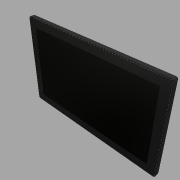
# Autodesk Inventor part: MageDok Screen
Saved by Autodesk Inventor 2019 (Build 230136000, 136)
## iProperties
Created: 2019-02-07
Part Number: MageDok Screen
Material: Generic
Document SubType Name: Modeling
Designer: Ben
Density: 1 g/cm^3
Appearance: Default
Author: Ben
Autodesk Inventor part; units mm, degrees
ref_plane "YZ Plane" through (0, 0, 0) normal (1, 0, 0) x (0, 1, 0)
ref_plane "XZ Plane" through (0, 0, 0) normal (0, 1, 0) x (-1, 0, 0)
sketch "Sketch1" plane through (0, 0, 0) normal (0, 0, 1) x (1, 0, 0)
  line L0 (152.5, -93.75) -> (-152.5, -93.75)
  line L1 (-152.5, -93.75) -> (-152.5, 93.75)
  line L2 (-152.5, 93.75) -> (152.5, 93.75)
  line L3 (152.5, 93.75) -> (152.5, -93.75)
  line L4 (152.5, -93.75) -> (-152.5, 93.75) construction
  line L5 (-152.5, -93.75) -> (152.5, 93.75) construction
  point P0 (0, 0)
  dimension "d0" = 305
  dimension "d1" = 187.5
  constraints: 12 end point, 2 midpoint, 2 parallel, 1 horizontal, 1 perpendicular
  measures "d0" distance of L1.end L2.end
  measures "d1" distance of L0.end L1.end
extrude "Extrusion1" add sketch "Sketch1" along normal blind 10.5
fillet "Fillet1" radius 4 4 edges at (152.5, 93.75, 5.25) (-152.5, 93.75, 5.25) (-152.5, -93.75, 5.25) (152.5, -93.75, 5.25)
chamfer "Chamfer1" distance 0.5 distance2 1 8 edges at (0, 93.75, 10.5) (-151.3284, 92.5784, 10.5) (-152.5, 0, 10.5) (-151.3284, -92.5784, 10.5) (0, -93.75, 10.5) (151.3284, -92.5784, 10.5) (152.5, 0, 10.5) (151.3284, 92.5784, 10.5) measured on face at (49.5, -31.25, 10.5)
chamfer "Chamfer2" distance 0.5 distance2 1.5 8 edges at (0, 93.75, 0) (151.3284, 92.5784, 0) (152.5, 0, 0) (151.3284, -92.5784, 0) (0, -93.75, 0) (-151.3284, -92.5784, 0) (-152.5, 0, 0) (-151.3284, 92.5784, 0) measured on face at (49.5, -31.25, 0)
sketch "Sketch2" plane through (0, 0, 10.5) normal (0, 0, 1) x (1, 0, 0)
  line L0 (-148.5, 93.25) -> (148.5, 93.25) construction
  arc A0 (-148.5, 93.25) -> (-152, 89.75) centre (-148.5, 89.75) ccw construction
  line L1 (-152, -89.75) -> (-152, 89.75) construction
  arc A1 (-152, -89.75) -> (-148.5, -93.25) centre (-148.5, -89.75) ccw construction
  line L2 (148.5, -93.25) -> (-148.5, -93.25) construction
  arc A2 (148.5, -93.25) -> (152, -89.75) centre (148.5, -89.75) ccw construction
  line L3 (152, 89.75) -> (152, -89.75) construction
  arc A3 (152, 89.75) -> (148.5, 93.25) centre (148.5, 89.75) ccw construction
  line L4 (148.5, 92.75) -> (-148.5, 92.75)
  arc A4 (-148.5, 92.75) -> (-151.5, 89.75) centre (-148.5, 89.75) ccw
  line L5 (-151.5, 89.75) -> (-151.5, -89.75)
  arc A5 (-151.5, -89.75) -> (-148.5, -92.75) centre (-148.5, -89.75) ccw
  line L6 (-148.5, -92.75) -> (148.5, -92.75)
  arc A6 (148.5, -92.75) -> (151.5, -89.75) centre (148.5, -89.75) ccw
  line L7 (151.5, -89.75) -> (151.5, 89.75)
  arc A7 (151.5, 89.75) -> (148.5, 92.75) centre (148.5, 89.75) ccw
  point P0 (0, 0)
  dimension "d11" = 0.5
  constraints: 8 end point, 8 point on circle, 4 centre point, 7 other
  measures "d11" distance between parallel lines of L0 L4
extrude "Extrusion2" cut sketch "Sketch2" against normal blind 0.25
fillet "Fillet2" radius 0.25 16 edges at (-150.6213, 91.8713, 10.5) (0, 92.75, 10.5) (150.6213, 91.8713, 10.5) (151.5, 0, 10.5) (150.6213, -91.8713, 10.5) (0, -92.75, 10.5) (-150.6213, -91.8713, 10.5) (-151.5, 0, 10.5) (0, 93.25, 10.5) (-150.9749, 92.2249, 10.5) (-152, 0, 10.5) (-150.9749, -92.2249, 10.5) (0, -93.25, 10.5) (150.9749, -92.2249, 10.5) (152, 0, 10.5) (150.9749, 92.2249, 10.5)
ref_plane "Work Plane1" through (0, 0, 10.5) normal (0, 0, 1) x (1, 0, 0)
sketch "Sketch3" plane through (0, 0, 10.5) normal (0, 0, 1) x (1, 0, 0)
  line L0 (-148.5, 92.75) -> (148.5, 92.75) projected
  arc A0 (-148.5, 92.75) -> (-151.5, 89.75) centre (-148.5, 89.75) ccw projected
  line L1 (-151.5, -89.75) -> (-151.5, 89.75) projected
  arc A1 (-151.5, -89.75) -> (-148.5, -92.75) centre (-148.5, -89.75) ccw projected
  line L2 (148.5, -92.75) -> (-148.5, -92.75) projected
  arc A2 (148.5, -92.75) -> (151.5, -89.75) centre (148.5, -89.75) ccw projected
  line L3 (151.5, 89.75) -> (151.5, -89.75) projected
  arc A3 (151.5, 89.75) -> (148.5, 92.75) centre (148.5, 89.75) ccw projected
  line L4 (-134.5, -75.75) -> (-134.5, 75.75)
  line L5 (-134.5, 75.75) -> (134.5, 75.75)
  line L6 (134.5, 75.75) -> (134.5, -75.75)
  line L7 (134.5, -75.75) -> (-134.5, -75.75)
  point P0 (0, 0)
  dimension "d16" = 17
  constraints: 8 end point, 3 other
  measures "d16" distance between parallel lines of L2 L7
extrude "Extrusion3" add sketch "Sketch3" against normal blind 1 separate body
sketch "Sketch4" plane through (0, 0, 10.5) normal (0, 0, 1) x (1, 0, 0)
  line L0 (-134.5, 75.75) -> (134.5, 75.75) projected
  line L1 (134.5, 75.75) -> (134.5, -75.75) projected
  line L2 (134.5, -75.75) -> (-134.5, -75.75) projected
  line L3 (-134.5, -75.75) -> (-134.5, 75.75) projected
  point P0 (0, 0)
extrude "Extrusion4" add sketch "Sketch4" against normal blind 1 separate body
sketch "Sketch5" plane through (152.5, -89.75, 9.5) normal (1, 0, 0) x (0, 0, -1)
  circle A0 centre (4, 11) radius 1.75
  circle A1 centre (4, 11) radius 2.5
  line L0 (0, -4) -> (8, -4) projected
  line L1 (8, 0) -> (0, 0) construction
  line L2 (4, 0) -> (4, 1) construction
  line L3 (4.575, 30.17) -> (3.425, 30.17)
  line L4 (2.675, 29.42) -> (2.675, 22.58)
  line L5 (3.425, 21.83) -> (4.575, 21.83)
  line L6 (5.325, 22.58) -> (5.325, 29.42)
  line L7 (5.325, 30.17) -> (2.675, 21.83) construction
  line L8 (2.675, 30.17) -> (5.325, 21.83) construction
  arc A2 (3.425, 30.17) -> (2.675, 29.42) centre (3.425, 29.42) ccw
  arc A3 (2.675, 22.58) -> (3.425, 21.83) centre (3.425, 22.58) ccw
  arc A4 (4.575, 21.83) -> (5.325, 22.58) centre (4.575, 22.58) ccw
  arc A5 (5.325, 29.42) -> (4.575, 30.17) centre (4.575, 29.42) ccw
  line L9 (3.65, 23) -> (4.35, 23)
  line L10 (4.35, 23) -> (4.35, 29)
  line L11 (4.35, 29) -> (3.65, 29)
  line L12 (3.65, 29) -> (3.65, 23)
  line L13 (3.65, 23) -> (4.35, 29) construction
  line L14 (4.35, 23) -> (3.65, 29) construction
  line L15 (5.25, 51.3) -> (3.75, 51.3)
  line L16 (3.75, 40.7) -> (5.25, 40.7)
  line L17 (5.25, 40.7) -> (5.25, 51.3)
  line L18 (5.25, 51.3) -> (3.75, 40.7) construction
  line L19 (3.75, 51.3) -> (5.25, 40.7) construction
  line L20 (2.75, 50.05) -> (2.75, 50.05)
  line L21 (2.75, 50.05) -> (2.75, 41.95)
  line L22 (2.75, 41.95) -> (2.75, 41.95)
  line L23 (2.75, 46) -> (3.7399, 45.8914) construction
  line L24 (3.75, 51.3) -> (3.75, 51.05)
  line L25 (3.75, 40.95) -> (3.75, 40.7)
  line L26 (2.75, 41.95) -> (3.75, 40.95)
  line L27 (2.75, 50.05) -> (3.75, 51.05)
  line L28 (5.25, 46) -> (2.75, 46) construction
  line L29 (4, 46) -> (4, 40) construction
  line L30 (5.425, 69.45) -> (4.275, 69.45)
  line L31 (3.575, 68.75) -> (3.575, 63.25)
  line L32 (4.275, 62.55) -> (5.425, 62.55)
  line L33 (5.425, 62.55) -> (5.425, 69.45)
  line L34 (5.425, 69.45) -> (3.575, 62.55) construction
  line L35 (3.575, 69.45) -> (5.425, 62.55) construction
  line L36 (4.275, 69.45) -> (3.575, 68.75)
  line L37 (4.275, 62.55) -> (3.575, 63.25)
  point P0 (9.5, 89.75)
  point P1 (4, 26)
  point P2 (4.5, 46)
  point P3 (3.75, 50.05)
  point P4 (3.75, 41.95)
  point P5 (4.5, 66)
  dimension "d21" = 3.5
  dimension "d22" = 5
  dimension "d23" = 15
  dimension "d24" = 1
  dimension "d25" = 0
  dimension "d26" = 2.65
  dimension "d27" = 8.34
  dimension "d28" = 15
  dimension "d29" = 0.75
  dimension "d30" = 0.7
  dimension "d31" = 6
  dimension "d32" = 0
  dimension "d45" = 1.5
  dimension "d46" = 10.6
  dimension "d47" = 1
  dimension "d48" = 8.1
  dimension "d50" = 1
  dimension "d51" = 1
  dimension "d52" = 1
  dimension "d53" = 1
  dimension "d54" = 1.25
  dimension "d55" = 1.5
  dimension "d56" = 20
  dimension "d58" = 0
  dimension "d59" = 1.85
  dimension "d60" = 6.9
  dimension "d61" = 20
  dimension "d62" = 0
  dimension "d63" = 0.7
  dimension "d64" = 0.7
  dimension "d65" = 0.7
  dimension "d66" = 0.7
  constraints: 72 end point, 16 point on line, 12 midpoint, 10 parallel, 8 point on circle, 8 tangent, 6 centre point, 6 perpendicular, 5 horizontal, 3 equal radius, 2 vertical, 1 coincident
  measures "d21" diameter of A0
  measures "d22" diameter of A1
  measures "d23" distance from line of L0 A0.centre
  measures "d24" distance of L2.start L2.end
  measures "d25" horizontal distance of L2.end A0.centre
  measures "d26" distance of L8.end L7.end
  measures "d27" distance of L7.end L8.start
  measures "d28" distance of A0.centre point (4, 26)
  measures "d29" radius of A2
  measures "d30" distance of L11.end L10.end
  measures "d31" distance of L10.end L9.end
  measures "d32" horizontal distance of A0.centre point (4, 26)
  measures "d45" distance of L16.end L16.start
  measures "d46" distance of L16.start L15.end
  measures "d47" distance of point (3.75, 41.95) L21.end
  measures "d48" distance of L21.end L20.end
  measures "d50" distance of L22.end point (3.75, 41.95)
  measures "d51" distance of L25.start point (3.75, 41.95)
  measures "d52" distance of L20.start point (3.75, 50.05)
  measures "d53" distance of L24.end point (3.75, 50.05)
  measures "d54" vertical distance of L15.end L20.end
  measures "d55" distance of L15.start L15.end
  measures "d56" vertical distance of point (4, 26) point (4.5, 46)
  measures "d58" horizontal distance of point (4, 26) L29.start
  measures "d59" distance of L32.end L34.end
  measures "d60" distance of L34.end L35.start
  measures "d61" vertical distance of L29.start point (4.5, 66)
  measures "d62" horizontal distance of point (4.5, 46) point (4.5, 66)
  measures "d63" distance of L30.end L35.start
  measures "d64" distance of L31.start L35.start
  measures "d65" distance of L32.start L34.end
  measures "d66" distance of L31.end L34.end
extrude "Extrusion5" cut sketch "Sketch5" against normal blind 5 contours A0 | A5 L6 A4 L5 A3 L4 A2 L3 | L12 L11 L10 L9 | L17 L16 L25 L26 L21 L27 L24 L15 | L33 L32 L37 L31 L36 L30 bodies 1
extrude "Extrusion6" add sketch "Sketch5" along normal blind 0.5 separate body contours A1
full round fillet "Fillet3" bodies 4 first side at (152.8333, -78.9512, 3.0081) centre faces at (153, -79.089, 3.2912) second side at (152.8333, -79.6853, 4.0209)
sketch "Sketch6" plane through (0, 0, 0) normal (0, 0, -1) x (-1, 0, 0)
  circle A0 centre (-143.325, 74.075) radius 3.175
  line L0 (-148.5, 93.25) -> (148.5, 93.25) construction
  line L1 (-152, -89.75) -> (-152, 89.75) construction
  circle A1 centre (-143.325, 66.225) radius 3.175
  circle A2 centre (-143.325, 58.375) radius 3.175
  circle A3 centre (-143.325, 50.525) radius 3.175
  circle A4 centre (-143.325, 41.175) radius 3.175
  point P0 (0, 0)
  dimension "d71" = 6.35
  dimension "d72" = 19.175
  dimension "d73" = 8.675
  dimension "d76" = 7.85
  dimension "d81" = 6.35
  dimension "d82" = 0
  dimension "d83" = 9.35
  constraints: 5 centre point, 1 vertical, 6 other
  measures "d71" diameter of A0
  measures "d72" distance from line of L0 A0.centre
  measures "d73" distance from line of L1 A0.centre
  measures "d76" distance of A0.centre A1.centre
  measures "d81" diameter of A4
  measures "d82" horizontal distance of A4.centre A0.centre
  measures "d83" distance of A3.centre A4.centre
extrude "Extrusion7" add sketch "Sketch6" along normal blind 1 separate body
equation "\"d48\" = d46 - 2.5 * d47"
equation "\"d50\" = d47"
equation "\"d51\" = d50"
equation "\"d52\" = d50"
equation "\"d53\" = d52"
equation "\"d54\" = -0.5 * d48 + 0.5 * d46"
equation "\"d55\" = d45"
equation "\"d61\" = d56"
equation "\"d64\" = d63"
equation "\"d65\" = d63"
equation "\"d66\" = d65"
equation "\"d81\" = d71"
body "Solid1"
body "Solid2"
body "Solid3"
body "Solid4"
body "Solid5"
